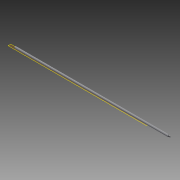
# Autodesk Inventor part: Rod
Saved by Autodesk Inventor 2015 (Build 190159000, 159)
## iProperties
Created: 2014-07-11
Part Number: Rod
Material: Generic
Document SubType Name: Modeling
Designer: jad211
Density: 1 g/cm^3
Appearance: Default
Author: jad211
Autodesk Inventor part; units mm, degrees
ref_plane "YZ Plane" through (0, 0, 0) normal (1, 0, 0) x (0, 1, 0)
ref_plane "XZ Plane" through (0, 0, 0) normal (0, 1, 0) x (-1, 0, 0)
sketch "Sketch1" plane through (0, 0, 0) normal (1, 0, 0) x (0, 1, 0)
  circle A0 centre (0, 0) radius 3
  dimension "d4" = 6
  constraints: 1 centre point
  measures "d4" diameter of A0
extrude "Extrusion1" add sketch "Sketch1" along normal blind 370
sketch "Sketch2" plane through (370, 0, 0) normal (1, 0, 0) x (0, 0, -1)
  circle A0 centre (0, 0) radius 2
  dimension "d5" = 4
  constraints: 1 centre point, 1 coincident
  measures "d5" diameter of A0
extrude "Extrusion2" add sketch "Sketch2" along normal blind 4
thread "Thread1" size "M4x0.7" class "6g" standard "ANSI Metric M Profile" full length
ref_plane "Work Plane1" through (0, 0, -3) normal (0, 0, 1) x (1, 0, 0)
sketch "Sketch3" plane through (0, 0, -3) normal (0, 0, 1) x (1, 0, 0)
  line L0 (374, 0.5) -> (368, 0.5)
  line L1 (368, 0.5) -> (368, -0.5)
  line L2 (368, -0.5) -> (374, -0.5)
  line L3 (374, -0.5) -> (374, 0.5)
  line L4 (374, 0.5) -> (368, -0.5) construction
  line L5 (368, 0.5) -> (374, -0.5) construction
  line L6 (374, -2) -> (374, 2) projected
  point P0 (0, 0)
  point P1 (371, 0)
  dimension "d10" = 1
  dimension "d11" = 6
  dimension "d18" = 0
  constraints: 12 end point, 3 perpendicular, 2 midpoint, 1 horizontal
  measures "d10" distance between parallel lines of L0 L2
  measures "d11" distance from line of L0.end L3
  measures "d18" distance between parallel lines of L6 L3
extrude "Extrusion3" cut sketch "Sketch3" along normal blind 1.5
sketch "Sketch4" plane through (0, 0, -3) normal (0, 0, 1) x (1, 0, 0)
  circle A0 centre (360, 0) radius 1
  line L0 (370, -3) -> (370, 3) projected
  point P0 (0, 0)
  point P1 (370, 0.5)
  point P2 (370, -0.5)
  dimension "d14" = 2
  dimension "d15" = 10
  constraints: 1 centre point
  measures "d14" diameter of A0
  measures "d15" distance from line of L0 A0.centre
extrude "Extrusion4" cut sketch "Sketch4" along normal up to next
body "Solid1"
